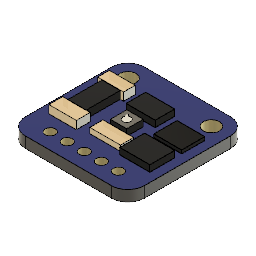
Case (Autodesk Fusion 360 archive; units mm, degrees)
design "SPG30 eCO2 sensor"
Autodesk Fusion 360 part; units mm, degrees
sketch "Sketch1" plane through (0, 0, 0) normal (0, 1, 0) x (1, 0, 0)
  line L0 (-0.857, 11.0235) -> (12.013, 11.0235)
  line L1 (14.513, 8.5235) -> (14.513, -4.3565)
  line L2 (12.013, -6.8565) -> (-0.857, -6.8565)
  line L3 (-3.357, -4.3565) -> (-3.357, 8.5235)
  circle A0 centre (-0.672, 8.3235) radius 1.2
  circle A1 centre (11.828, 8.3235) radius 1.2
  line L4 (4.353, 3.1235) -> (6.803, 3.1235)
  line L5 (6.803, 3.1235) -> (6.803, 0.6735)
  line L6 (6.803, 0.6735) -> (4.353, 0.6735)
  line L7 (4.353, 0.6735) -> (4.353, 3.1235)
  circle A2 centre (5.578, -4.4565) radius 0.75
  line L8 (-3.357, -4.4565) -> (14.513, -4.4565)
  circle A3 centre (8.128, -4.4565) radius 0.75
  circle A4 centre (10.678, -4.4565) radius 0.75
  circle A5 centre (3.028, -4.4565) radius 0.75
  circle A6 centre (0.478, -4.4565) radius 0.75
  arc A7 (-0.857, 11.0235) -> (-3.357, 8.5235) centre (-0.857, 8.5235) ccw
  arc A8 (14.513, 8.5235) -> (12.013, 11.0235) centre (12.013, 8.5235) ccw
  arc A9 (12.013, -6.8565) -> (14.513, -4.3565) centre (12.013, -4.3565) ccw
  arc A10 (-3.357, -4.3565) -> (-0.857, -6.8565) centre (-0.857, -4.3565) ccw
  line L9 (5.578, 11.0235) -> (5.578, -6.8565)
  line L10 (-0.672, 8.3235) -> (11.828, 8.3235)
  dimension "d1" = 2.4
  dimension "d4" = 17.88
  dimension "d5" = 2.7
  dimension "d6" = 2.7
  dimension "d7" = 2.45
  dimension "d8" = 2.45
  dimension "d12" = 1.5
  dimension "d13" = 2.4
  dimension "d18" = 2.55
  dimension "d19" = 2.55
  dimension "d20" = 2.55
  dimension "d21" = 2.55
  dimension "d22" = 2.5
  dimension "d27" = 5.2
  dimension "d51" = 12.5
  dimension "d52" = 17.87
  measures "d1" diameter of A0
  measures "d4" distance of L0 L2
  measures "d5" distance of L0
  measures "d6" distance of L0
  measures "d12" diameter of A2
  measures "d13" distance of L2 L8
  measures "d22" radius of A7
  measures "d27" distance of L4
  measures "d52" distance of L1 L3
extrude "Extrude1" add sketch "Sketch1" along normal blind 1.65 contours L0 L3 L4 L6 L7 A2 L8 A5 A6 A7 A10 L9 | L0 L1 L4 L5 L6 A2 L8 A3 A4 A8 A9 L9 | L2 A2 L8 A5 A6 A10 L9 | L2 A2 L8 A3 A4 A9 L9
extrude "Extrude2" add sketch "Sketch1" along normal blind 2.65 contours L4 L6 L7 L9 | L4 L5 L6 L9
sketch "Sketch2" plane through (0, 1.65, 0) normal (0, 1, 0) x (-1, 0, 0)
  circle A0 centre (-5.578, 4.4565) radius 0.75
  circle A1 centre (-0.478, 4.4565) radius 0.75
  circle A2 centre (0.672, -8.3235) radius 1.2
  circle A3 centre (-10.678, 4.4565) radius 0.75
  circle A4 centre (-8.128, 4.4565) radius 0.75
  line L0 (-6.803, -0.6735) -> (-4.353, -0.6735)
  line L1 (-4.353, -0.6735) -> (-4.353, -3.1235)
  line L2 (-4.353, -3.1235) -> (-6.803, -3.1235)
  line L3 (-6.803, -3.1235) -> (-6.803, -0.6735)
  circle A5 centre (-3.028, 4.4565) radius 0.75
  circle A6 centre (-11.828, -8.3235) radius 1.2
  arc A7 (0.857, -11.0235) -> (3.357, -8.5235) centre (0.857, -8.5235) ccw
  line L4 (3.357, -8.5235) -> (3.357, 4.3565)
  arc A8 (3.357, 4.3565) -> (0.857, 6.8565) centre (0.857, 4.3565) ccw
  line L5 (0.857, 6.8565) -> (-12.013, 6.8565)
  arc A9 (-12.013, 6.8565) -> (-14.513, 4.3565) centre (-12.013, 4.3565) ccw
  line L6 (-14.513, 4.3565) -> (-14.513, -8.5235)
  arc A10 (-14.513, -8.5235) -> (-12.013, -11.0235) centre (-12.013, -8.5235) ccw
  line L7 (-12.013, -11.0235) -> (0.857, -11.0235)
  line L8 (1.8732, -6.733) -> (-2, -6.733)
  line L9 (-2, -6.733) -> (-2, -5)
  line L10 (-2, -5) -> (1.8732, -5)
  line L11 (1.8732, -5) -> (1.8732, -6.733)
  line L12 (1.2394, -5) -> (-1.5006, -5)
  line L13 (-1.5006, -5) -> (-1.5006, 0.1577)
  line L14 (-1.5006, 0.1577) -> (1.2394, 0.1577)
  line L15 (1.2394, 0.1577) -> (1.2394, -5)
  line L16 (1.955, 0.1577) -> (-2.1549, 0.1577)
  line L17 (-2.1549, 0.1577) -> (-2.1549, 2.2229)
  line L18 (-2.1549, 2.2229) -> (1.955, 2.2229)
  line L19 (1.955, 2.2229) -> (1.955, 0.1577)
  line L20 (-3.6884, -0.224) -> (-8.2686, -0.224)
  line L21 (-8.2686, -0.224) -> (-8.2686, 1.731)
  line L22 (-8.2686, 1.731) -> (-3.6884, 1.731)
  line L23 (-3.6884, 1.731) -> (-3.6884, -0.224)
  line L24 (-3.4431, -3.9317) -> (-7.7984, -3.9317)
  line L25 (-7.7984, -3.9317) -> (-7.7984, -6.8557)
  line L26 (-7.7984, -6.8557) -> (-3.4431, -6.8557)
  line L27 (-3.4431, -6.8557) -> (-3.4431, -3.9317)
  line L28 (-9, -6) -> (-13.176, -6)
  line L29 (-13.176, -6) -> (-13.176, -2.5209)
  line L30 (-13.176, -2.5209) -> (-9, -2.5209)
  line L31 (-9, -2.5209) -> (-9, -6)
  line L32 (-8.6776, -1.4781) -> (-13.176, -1.4781)
  line L33 (-13.176, -1.4781) -> (-13.176, 2.2433)
  line L34 (-13.176, 2.2433) -> (-8.6776, 2.2433)
  line L35 (-8.6776, 2.2433) -> (-8.6776, -1.4781)
extrude "Extrude3" add sketch "Sketch2" along normal blind 1.2 contours L8 L9 L10 L11 L12 | L14 L16 L17 L18 L19
extrude "Extrude4" add sketch "Sketch2" along normal blind 0.97 contours L24 L25 L26 L27 | L32 L33 L34 L35
extrude "Extrude5" add sketch "Sketch2" along normal blind 0.5 contours L28 L29 L30 L31
extrude "Extrude6" add sketch "Sketch2" along normal blind 1.15 contours L10 L12 L13 L14 L15 L16
extrude "Extrude7" add sketch "Sketch2" along normal blind 0.81 contours L20 L21 L22 L23
sketch "Sketch3" plane through (0, 2.65, 0) normal (0, 1, 0) x (-1, 0, 0)
  line L0 (-4.353, -0.6735) -> (-6.803, -0.6735)
  line L1 (-6.803, -0.6735) -> (-6.803, -3.1235)
  line L2 (-6.803, -3.1235) -> (-4.353, -3.1235)
  line L3 (-4.353, -3.1235) -> (-4.353, -0.6735)
  circle A0 centre (-5.578, -1.8985) radius 0.58
  line L4 (-5.578, -3.1235) -> (-5.578, -0.6735)
  line L5 (-5.578, -1.8985) -> (-4.9008, -2.5757)
  line L6 (-5.578, -1.8985) -> (-4.4704, -1.8985) construction
  line L7 (-4.9008, -2.5757) -> (-5.0253, -2.7001)
  line L8 (-5.0253, -2.7001) -> (-5.3117, -2.4137)
  line L9 (-4.9008, -2.5757) -> (-4.7764, -2.4512)
  line L10 (-4.7764, -2.4512) -> (-5.0628, -2.1648)
  dimension "d44" = 1.16
  dimension "d45" = 45
  measures "d44" diameter of A0
  measures "d45" angle of L5 L6
extrude "Extrude8" cut sketch "Sketch3" against normal blind 0.01 contours A0 L4 | A0 L4 L5 | A0 L4 L5 | A0 L5 L9 L10 | A0 L5 L7 L8
equation "d5 = 1.5 mm + ( ( 2.4 / 2 ) * 1 mm )"
equation "d27 = 4.0 mm + ( ( 2.4 / 2 ) * 1 mm )"
equation "d34 = 2.85 mm - 1.65 mm"
equation "d36 = 2.62 mm - 1.65 mm"
equation "d38 = 2.15 mm - 1.65 mm"
equation "d40 = 2.8 mm - 1.65 mm"
equation "d42 = 2.46 mm - 1.65 mm"

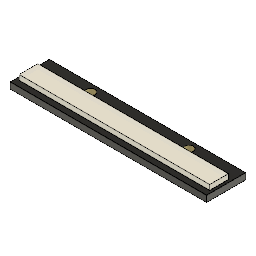
design "NeoPixel bar"
Autodesk Fusion 360 part; units mm, degrees
sketch "Sketch1" plane through (0, 0, 0) normal (0, 1, 0) x (1, 0, 0)
  line L0 (-25.528, 5.5699) -> (25.272, 5.5699)
  line L1 (25.272, 5.5699) -> (25.272, -4.5901)
  line L2 (25.272, -4.5901) -> (-25.528, -4.5901)
  line L3 (-25.528, -4.5901) -> (-25.528, 5.5699)
  circle A0 centre (-12.828, 3.5379) radius 1.14
  circle A1 centre (12.572, 3.5379) radius 1.14
  line L4 (-24.725, 1.7545) -> (24.551, 1.7545)
  line L5 (24.551, 1.7545) -> (24.551, -3.0715)
  line L6 (24.551, -3.0715) -> (-24.725, -3.0715)
  line L7 (-24.725, -3.0715) -> (-24.725, 1.7545)
  line L8 (-26.6596, 3.5379) -> (-26.3085, 3.5379)
  line L9 (-26.3085, 3.5379) -> (27.3498, 3.5379)
  dimension "d1" = 50.8
  dimension "d2" = 10.16
  dimension "d3" = 2.28
  dimension "d5" = 49.276
  dimension "d6" = 4.826
  dimension "d11" = 8.128
  dimension "d12" = 12.7
  dimension "d13" = 38.1
  measures "d3" diameter of A0
  measures "d11" distance of L9
  measures "d12" distance of L3
  measures "d13" distance of L3
extrude "Extrude1" add sketch "Sketch1" along normal blind 2.95 contours L4 L5 L6 L7
extrude "Extrude2" add sketch "Sketch1" along normal blind 1.65 contours L0 L1 L3 A0 A1 L9 | L1 L2 L3 A0 A1 L9
sketch "Sketch2" plane through (0, 0, 0) normal (0, -1, 0) x (1, 0, 0)
  line L0 (25.272, 4.5901) -> (-25.528, 4.5901)
  line L1 (-25.528, 4.5901) -> (-25.528, -5.5699)
  line L2 (-25.528, -5.5699) -> (25.272, -5.5699)
  line L3 (25.272, -5.5699) -> (25.272, 4.5901)
  circle A0 centre (-12.828, -3.5379) radius 1.14
  circle A1 centre (12.572, -3.5379) radius 1.14
  line L4 (-22.028, 9.0432) -> (-22.028, -12.1187)
  line L5 (21.772, 13.1512) -> (21.772, -13.5403)
  line L6 (25.272, -5.5699) -> (25.272, 4.5901)
  line L7 (-25.528, 4.5901) -> (-25.528, -5.5699)
  dimension "d14" = 3.5
  dimension "d15" = 3.5
  measures "d14" distance of L5 L6
  measures "d15" distance of L4 L7
split_face "SplitFace1" 1 faces at (-4.2225, 0, 2.2345) by curves path "Sketch2" along L4
split_face "SplitFace2" 1 faces at (5.1874, 0, 2.2513) by curves path "Sketch2" along L5
equation "d7 = 1.65 mm + 1.3 mm"

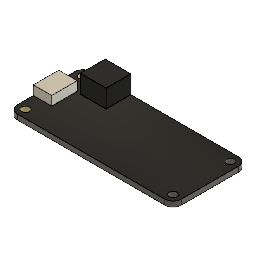
design "Feather M0"
Autodesk Fusion 360 part; units mm, degrees
sketch "Sketch1" plane through (0, 0, 0) normal (0, 1, 0) x (1, 0, 0)
  line L0 (2.4136, 23.4111) -> (48.1336, 23.4111)
  line L1 (50.6736, 20.8711) -> (50.6736, 3.0911)
  line L2 (48.1336, 0.5511) -> (2.4136, 0.5511)
  line L3 (-0.1264, 3.0911) -> (-0.1264, 20.8711)
  circle A0 centre (2.4136, 20.8711) radius 1.2
  circle A1 centre (2.4212, 3.0911) radius 1.2
  circle A2 centre (48.1336, 3.0911) radius 1.2
  circle A3 centre (48.1336, 20.8711) radius 1.2
  arc A4 (2.4136, 23.4111) -> (-0.1264, 20.8711) centre (2.4136, 20.8711) ccw
  arc A5 (-0.1264, 3.0911) -> (2.4136, 0.5511) centre (2.4136, 3.0911) ccw
  arc A6 (48.1336, 0.5511) -> (50.6736, 3.0911) centre (48.1336, 3.0911) ccw
  arc A7 (50.6736, 20.8711) -> (48.1336, 23.4111) centre (48.1336, 20.8711) ccw
  dimension "d1" = 50.8
  dimension "d2" = 22.86
  dimension "d3" = 2.4
  dimension "d4" = 2.54
  dimension "d5" = 2.54
  dimension "d6" = 45.72
  dimension "d7" = 17.78
  dimension "d8" = 2.54
  dimension "d9" = 2.54
  dimension "d10" = 2.54
  dimension "d11" = 2.5476
  dimension "d12" = 2.54
  measures "d3" diameter of A0
  measures "d4" distance of L0
  measures "d5" distance of L3
  measures "d6" distance of origin
  measures "d7" distance of origin
  measures "d8" distance of L0 origin
  measures "d9" distance of L1
  measures "d10" distance of L2
  measures "d11" distance of L3
  measures "d12" radius of A4
extrude "Extrude1" add sketch "Sketch1" along normal blind 1.65
sketch "Sketch2" plane through (0, 1.65, 0) normal (0, 1, 0) x (-1, 0, 0)
  circle A0 centre (-2.4212, -3.0911) radius 1.2
  circle A1 centre (-48.1336, -20.8711) radius 1.2
  circle A2 centre (-48.1336, -3.0911) radius 1.2
  circle A3 centre (-2.4136, -20.8711) radius 1.2
  arc A4 (-48.1336, -0.5511) -> (-50.6736, -3.0911) centre (-48.1336, -3.0911) ccw
  line L0 (-50.6736, -3.0911) -> (-50.6736, -20.8711)
  arc A5 (-50.6736, -20.8711) -> (-48.1336, -23.4111) centre (-48.1336, -20.8711) ccw
  line L1 (-48.1336, -23.4111) -> (-2.4136, -23.4111)
  arc A6 (-2.4136, -23.4111) -> (0.1264, -20.8711) centre (-2.4136, -20.8711) ccw
  line L2 (0.1264, -20.8711) -> (0.1264, -3.0911)
  arc A7 (0.1264, -3.0911) -> (-2.4136, -0.5511) centre (-2.4136, -3.0911) ccw
  line L3 (-2.4136, -0.5511) -> (-48.1336, -0.5511)
  line L4 (0.1264, -15.9435) -> (-5.5886, -15.9435)
  line L5 (-5.5886, -15.9435) -> (-5.5886, -8.0187)
  line L6 (-5.5886, -8.0187) -> (0.1264, -8.0187)
  line L7 (0.1264, -8.0187) -> (0.1264, -15.9435)
  line L8 (-6.7951, -23.4111) -> (-14.7961, -23.4111)
  line L9 (-14.7961, -23.4111) -> (-14.7961, -15.6641)
  line L10 (-14.7961, -15.6641) -> (-6.7951, -15.6641)
  line L11 (-6.7951, -15.6641) -> (-6.7951, -23.4111)
  dimension "d15" = 5.715
  dimension "d16" = 7.9248
  dimension "d17" = 8.001
  dimension "d18" = 7.747
  dimension "d19" = 10.922
  measures "d19" distance of L2
extrude "Extrude2" add sketch "Sketch2" along normal blind 5.588 contours L1 L8 L9 L10 L11
split_face "SplitFace1" 1 faces at (9.4621, 3.5127, -23.4111) by curves path "Sketch2" along L9 L10 L11 L8
extrude "Extrude3" add sketch "Sketch2" along normal blind 2.8448 contours L2 L4 L5 L6 L7
split_face "SplitFace2" 1 faces at (-0.1264, 2.5983, -13.3019) by curves path "Sketch2" along L4 L5 L6 L7
equation "d20 = 0.285 in - 0.065 in"
equation "d22 = 0.177 in - 0.065 in"
